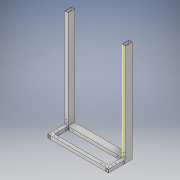
# Autodesk Inventor part: battery shelf frame
Saved by Autodesk Inventor 2018 (Build 220112000, 112)
## iProperties
Created: 2018-12-12
Part Number: battery shelf frame
Material: Generic
Document SubType Name: Modeling
Designer: s-4008082
Density: 1 g/cm^3
Appearance: Default
Author: s-4008082
Autodesk Inventor part; units mm, degrees
ref_plane "YZ Plane" through (0, 0, 0) normal (1, 0, 0) x (0, 1, 0)
ref_plane "XZ Plane" through (0, 0, 0) normal (0, 1, 0) x (-1, 0, 0)
ref_plane "XY Plane" through (0, 0, 0) normal (0, 0, 1) x (1, 0, 0)
sketch "Sketch1" plane through (0, 0, 0) normal (0, 1, 0) x (-1, 0, 0)
  line L0 (0, 0) -> (25.4, 0)
  line L1 (25.4, 0) -> (25.4, 50.8)
  line L2 (25.4, 50.8) -> (0, 50.8)
  line L3 (0, 50.8) -> (0, 0)
  line L4 (22.86, 48.26) -> (2.54, 48.26)
  line L5 (2.54, 48.26) -> (2.54, 2.54)
  line L6 (2.54, 2.54) -> (22.86, 2.54)
  line L7 (22.86, 2.54) -> (22.86, 48.26)
  dimension "d0" = 50.8
  dimension "d1" = 25.4
  dimension "d2" = 2.54
  dimension "d3" = 2.54
  dimension "d4" = 2.54
  dimension "d5" = 2.54
  constraints: 16 end point, 4 parallel, 2 horizontal, 2 perpendicular
  measures "d0" distance of L0.end L1.end
  measures "d1" distance of L1.end L2.end
  measures "d2" distance between parallel lines of L0 L6
  measures "d3" distance between parallel lines of L3 L5
  measures "d4" distance between parallel lines of L2 L4
  measures "d5" distance between parallel lines of L1 L7
extrude "Extrusion1" add sketch "Sketch1" along normal blind 762
sketch "Sketch2" plane through (0, 0, 50.8) normal (1, 0, 0) x (0, 0, -1)
  line L0 (0, 0) -> (50.8, 0) projected
  line L1 (0, 0) -> (0, 762) projected
  line L2 (50.8, 0) -> (0, 0)
  line L3 (0, 0) -> (0, 25.4)
  line L4 (0, 25.4) -> (50.8, 25.4)
  line L5 (50.8, 25.4) -> (50.8, 0)
  line L6 (48.26, 0) -> (48.26, 762) projected
  line L7 (2.54, 0) -> (2.54, 762) projected
  line L8 (48.26, 2.54) -> (2.54, 2.54)
  line L9 (2.54, 2.54) -> (2.54, 22.86)
  line L10 (2.54, 22.86) -> (48.26, 22.86)
  line L11 (48.26, 22.86) -> (48.26, 2.54)
  dimension "d8" = 25.4
  dimension "d9" = 2.54
  dimension "d10" = 2.54
  constraints: 16 end point, 4 parallel, 3 point on line, 2 horizontal, 2 perpendicular
  measures "d8" distance of L4.end L0.end
  measures "d9" distance between parallel lines of L4 L10
  measures "d10" distance between parallel lines of L8 L0
extrude "Extrusion2" add sketch "Sketch2" along normal blind 406.4 contours L1 L4 L7 L0 | L7 L8 L6 L0 | L6 L4 L5 L0 | L4 L6 L10 L7
sketch "Sketch3" plane through (-25.4, 762, 50.8) normal (0, 0, 1) x (1, 0, 0)
  point P0 (25.4, -762)
sketch "Sketch4" plane through (0, 0, 0) normal (0, -1, 0) x (1, 0, 0)
  line L0 (0, 0) -> (406.4, 0) projected
  line L1 (406.4, 0) -> (431.8, 0)
  line L2 (431.8, 0) -> (431.8, 50.8)
  line L3 (431.8, 50.8) -> (406.4, 50.8)
  line L4 (406.4, 50.8) -> (406.4, 0)
  line L5 (408.94, 48.26) -> (429.26, 48.26)
  line L6 (429.26, 48.26) -> (429.26, 2.54)
  line L7 (429.26, 2.54) -> (408.94, 2.54)
  line L8 (408.94, 2.54) -> (408.94, 48.26)
  dimension "d13" = 25.4
  dimension "d14" = 2.54
  dimension "d15" = 2.54
  dimension "d16" = 2.54
  dimension "d17" = 2.54
  constraints: 16 end point, 4 parallel, 2 horizontal, 2 perpendicular
  measures "d13" distance of L2.end L3.end
  measures "d14" distance between parallel lines of L3 L5
  measures "d15" distance between parallel lines of L2 L6
  measures "d16" distance between parallel lines of L1 L7
  measures "d17" distance between parallel lines of L8 L4
extrude "Extrusion3" add sketch "Sketch4" against normal blind 762
sketch "Sketch6" plane through (-25.4, 0, 0) normal (0, 0, -1) x (-1, 0, 0)
  circle A0 centre (-12.7, 12.7) radius 2.5797
  line L0 (0, 0) -> (0, 762) projected
  line L1 (-457.2, 0) -> (0, 0) projected
  circle A1 centre (-12.7, 38.1) radius 2.5797
  circle A2 centre (-12.7, 63.5) radius 2.5797
  circle A3 centre (-38.1, 13.2387) radius 2.5797
  circle A4 centre (-63.5, 12.7) radius 2.5797
  circle A5 centre (-12.7, 12.7) radius 2.5797
  line L2 (0, 0) -> (0, 762)
  line L3 (-457.2, 0) -> (0, 0)
  circle A6 centre (-12.7, 38.1) radius 2.5797
  circle A7 centre (-12.7, 63.5) radius 2.5797
  circle A8 centre (-38.1, 13.2387) radius 2.5797
  circle A9 centre (-63.5, 12.7) radius 2.5797
  line L4 (-25.4, 2.54) -> (-431.8, 2.54) projected
  line L5 (-228.6, 2.54) -> (-228.6, 762)
  circle A10 centre (-444.5, 12.7) radius 2.5797
  circle A11 centre (-444.5, 38.1) radius 2.5797
  circle A12 centre (-419.1, 13.2387) radius 2.5797
  circle A13 centre (-393.7, 12.7) radius 2.5797
  circle A14 centre (-444.5, 63.5) radius 2.5797
  point P0 (-25.4, 0)
  point P1 (-25.4, 0)
  dimension "d22" = 12.7
  dimension "d23" = 12.7
  dimension "d24" = 5.1594
  dimension "d25" = 25.4
  dimension "d26" = 5.1594
  dimension "d27" = 25.4
  dimension "d28" = 5.1594
  dimension "d29" = 25.4
  dimension "d30" = 5.1594
  dimension "d31" = 12.7
  dimension "d32" = 5.1594
  dimension "d33" = 25.4
  dimension "d36" = 12.7
  dimension "d37" = 12.7
  dimension "d38" = 5.1594
  dimension "d39" = 25.4
  dimension "d40" = 5.1594
  dimension "d41" = 25.4
  dimension "d42" = 5.1594
  dimension "d43" = 25.4
  dimension "d44" = 5.1594
  dimension "d45" = 12.7
  dimension "d46" = 5.1594
  dimension "d47" = 25.4
  constraints: 15 centre point, 6 end point, 5 symmetric about line, 1 midpoint, 1 perpendicular, 5 other
  measures "d22" distance from line of L0 A0.centre
  measures "d23" distance from line of L1 A0.centre
  measures "d24" diameter of A0
  measures "d25" distance of A0.centre A1.centre
  measures "d26" diameter of A1
  measures "d27" distance of A1.centre A2.centre
  measures "d28" diameter of A2
  measures "d29" horizontal distance of A0.centre A3.centre
  measures "d30" diameter of A3
  measures "d31" distance from line of L1 A4.centre
  measures "d32" diameter of A4
  measures "d33" horizontal distance of A3.centre A4.centre
  measures "d36" distance from line of L2 A5.centre
  measures "d37" distance from line of L3 A5.centre
  measures "d38" diameter of A5
  measures "d39" distance of A5.centre A6.centre
  measures "d40" diameter of A6
  measures "d41" distance of A6.centre A7.centre
  measures "d42" diameter of A7
  measures "d43" horizontal distance of A5.centre A8.centre
  measures "d44" diameter of A8
  measures "d45" distance from line of L3 A9.centre
  measures "d46" diameter of A9
  measures "d47" horizontal distance of A8.centre A9.centre
extrude "Extrusion6" cut sketch "Sketch6" against normal blind 736.6
sketch "Sketch8" plane through (-25.4, 0, 50.8) normal (0, 0, 1) x (1, 0, 0)
  line L0 (25.4, 25.4) -> (25.4, 762) projected
  line L1 (0, 0) -> (25.4, 0)
  line L2 (25.4, 0) -> (25.4, 25.4)
  line L3 (25.4, 25.4) -> (0, 25.4)
  line L4 (0, 25.4) -> (0, 0)
  line L5 (2.54, 2.54) -> (22.86, 2.54)
  line L6 (22.86, 2.54) -> (22.86, 22.86)
  line L7 (22.86, 22.86) -> (2.54, 22.86)
  line L8 (2.54, 22.86) -> (2.54, 2.54)
  line L9 (0, 0) -> (457.2, 0) projected
  point P0 (25.4, 0)
  dimension "d50" = 25.4
  dimension "d51" = 2.54
  dimension "d52" = 0
  dimension "d53" = 2.54
  dimension "d54" = 2.54
  dimension "d55" = 2.54
  constraints: 16 end point, 4 parallel, 2 horizontal, 2 perpendicular, 1 point on line
  measures "d50" distance of L3.end L1.start
  measures "d51" distance between parallel lines of L3 L7
  measures "d52" distance between parallel lines of L9 L1
  measures "d53" distance between parallel lines of L5 L1
  measures "d54" distance between parallel lines of L2 L6
  measures "d55" distance between parallel lines of L4 L8
extrude "Extrusion7" add sketch "Sketch8" along normal blind 127
sketch "Sketch10" plane through (406.4, 762, 50.8) normal (0, 0, 1) x (1, 0, 0)
  line L0 (0, -736.6) -> (0, 0) projected
  line L1 (0, -736.6) -> (0, -762)
  point P0 (-406.4, -762)
  constraints: 2 end point, 1 vertical
sketch "Sketch11" plane through (406.4, 762, 50.8) normal (0, 0, 1) x (1, 0, 0)
  line L0 (-406.4, -762) -> (-406.4, -736.6) projected
  line L1 (-406.4, -762) -> (-406.4, -736.6)
  constraints: 2 end point, 1 vertical
sketch "Sketch12" plane through (406.4, 762, 50.8) normal (0, 0, 1) x (1, 0, 0)
  line L0 (0, -736.6) -> (0, 0) projected
  line L1 (25.4, -762) -> (25.4, 0) projected
  line L2 (0, -736.6) -> (25.4, -736.6)
  line L3 (25.4, -736.6) -> (25.4, -762)
  line L4 (25.4, -762) -> (0, -762)
  line L5 (0, -762) -> (0, -736.6)
  line L6 (22.86, -762) -> (22.86, 0) projected
  line L7 (22.86, -739.14) -> (2.54, -739.14)
  line L8 (2.54, -739.14) -> (2.54, -759.46)
  line L9 (2.54, -759.46) -> (22.86, -759.46)
  line L10 (22.86, -759.46) -> (22.86, -739.14)
  point P0 (-406.4, -762)
  dimension "d62" = 2.54
  dimension "d63" = 2.54
  dimension "d64" = 2.54
  constraints: 16 end point, 4 parallel, 2 horizontal, 2 perpendicular, 1 point on line
  measures "d62" distance between parallel lines of L5 L8
  measures "d63" distance between parallel lines of L2 L7
  measures "d64" distance between parallel lines of L4 L9
extrude "Extrusion9" add sketch "Sketch12" along normal blind 127 contours L4 L6 L2 L1 | L4 L5 L2 L6 L7 L8 L9
sketch "Sketch9" plane through (-25.4, 0, 0) normal (-1, 0, 0) x (0, 0, 1)
  circle A0 centre (64.7925, 12.7) radius 9.525
  line L0 (0, 0) -> (177.8, 0) projected
  dimension "d58" = 19.05
  dimension "d59" = 12.7
  constraints: 1 centre point
  measures "d58" diameter of A0
  measures "d59" distance from line of L0 A0.centre
extrude "Extrusion8" cut sketch "Sketch9" against normal blind 508
sketch "Sketch13" plane through (0, 0, 50.8) normal (1, 0, 0) x (0, 0, -1)
  line L0 (-127, 0) -> (-101.6, 0)
  line L1 (-101.6, 0) -> (-101.6, 25.4)
  line L2 (-101.6, 25.4) -> (-127, 25.4)
  line L3 (-127, 25.4) -> (-127, 0)
  line L4 (0, 0) -> (-127, 0) projected
  line L5 (-127, 0) -> (-127, 25.4) projected
  line L6 (0, 2.54) -> (-127, 2.54) projected
  line L7 (-104.14, 2.54) -> (-124.46, 2.54)
  line L8 (-124.46, 2.54) -> (-124.46, 22.86)
  line L9 (-124.46, 22.86) -> (-104.14, 22.86)
  line L10 (-104.14, 22.86) -> (-104.14, 2.54)
  point P0 (50.8, 0)
  dimension "d67" = 25.4
  dimension "d68" = 25.4
  dimension "d69" = 0
  dimension "d70" = 0
  dimension "d71" = 2.54
  dimension "d72" = 2.54
  dimension "d73" = 2.54
  constraints: 16 end point, 4 parallel, 2 horizontal, 2 perpendicular, 1 point on line
  measures "d67" distance of L1.end L2.end
  measures "d68" distance of L2.end L0.start
  measures "d69" distance between parallel lines of L4 L0
  measures "d70" distance between parallel lines of L5 L3
  measures "d71" distance between parallel lines of L3 L8
  measures "d72" distance between parallel lines of L2 L9
  measures "d73" distance between parallel lines of L1 L10
extrude "Extrusion10" add sketch "Sketch13" along normal blind 406.4 contours L3 L6 L1 L0 | L3 L2 L1 L6 L10 L9 L8
sketch "Sketch14" plane through (-25.4, 25.4, 50.8) normal (0, 1, 0) x (1, 0, 0)
  line L0 (457.2, -127) -> (0, -127) projected
  line L1 (228.6, -127) -> (228.6, 50.8)
  line L2 (25.4, 50.8) -> (431.8, 50.8) projected
  circle A0 centre (444.5, -114.3) radius 2.5797
  circle A1 centre (419.1, -114.3) radius 2.5797
  circle A2 centre (393.7, -114.3) radius 2.5797
  circle A3 centre (444.5, -88.9) radius 2.5797
  circle A4 centre (444.5, -63.5) radius 2.5797
  line L3 (457.2, 0) -> (457.2, -127) projected
  circle A5 centre (12.7, -114.3) radius 2.5797
  circle A6 centre (38.1, -114.3) radius 2.5797
  circle A7 centre (63.5, -114.3) radius 2.5797
  circle A8 centre (12.7, -88.9) radius 2.5797
  circle A9 centre (12.7, -63.5) radius 2.5797
  dimension "d76" = 90
  dimension "d77" = 228.6
  dimension "d78" = 12.7
  dimension "d79" = 12.7
  dimension "d80" = 12.7
  dimension "d81" = 12.7
  dimension "d82" = 12.7
  dimension "d83" = 12.7
  dimension "d84" = 5.1594
  dimension "d85" = 5.1594
  dimension "d86" = 5.1594
  dimension "d87" = 5.1594
  dimension "d88" = 5.1594
  dimension "d89" = 25.4
  dimension "d90" = 25.4
  dimension "d91" = 25.4
  dimension "d92" = 25.4
  constraints: 10 centre point, 10 symmetric about line, 2 end point, 2 midpoint, 5 other
  measures "d76" angle of L0 L1
  measures "d77" distance from line of L1 L0.start
  measures "d78" distance from line of L3 A4.centre
  measures "d79" distance from line of L3 A3.centre
  measures "d80" distance from line of L3 A0.centre
  measures "d81" distance from line of L0 A0.centre
  measures "d82" distance from line of L0 A1.centre
  measures "d83" distance from line of L0 A2.centre
  measures "d84" diameter of A0
  measures "d85" diameter of A1
  measures "d86" diameter of A2
  measures "d87" diameter of A3
  measures "d88" diameter of A4
  measures "d89" distance of A3.centre A0.centre
  measures "d90" distance of A3.centre A4.centre
  measures "d91" distance of A1.centre A0.centre
  measures "d92" distance of A1.centre A2.centre
extrude "Extrusion11" cut sketch "Sketch14" against normal blind 406.4
body "Solid1"
